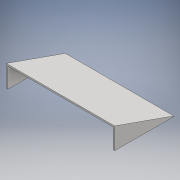
# Autodesk Inventor part: Front_Chassi
Saved by Autodesk Inventor 2018.2 (Build 222227000, 227)
## iProperties
Created: 2018-08-12
Part Number: Front_Chassi
Material: Generic
Document SubType Name: Modeling
Designer: mateu
Density: 1 g/cm^3
Appearance: Default
Author: mateu
Autodesk Inventor part; units mm, degrees
ref_plane "YZ Plane" through (0, 0, 0) normal (1, 0, 0) x (0, 1, 0)
ref_plane "XZ Plane" through (0, 0, 0) normal (0, 1, 0) x (-1, 0, 0)
ref_plane "XY Plane" through (0, 0, 0) normal (0, 0, 1) x (1, 0, 0)
sketch "Sketch1" plane through (0, 0, 0) normal (0, 0, 1) x (1, 0, 0)
  line L0 (0, 0) -> (0, 85)
  line L1 (0, 85) -> (156, 85)
  line L2 (156, 85) -> (156, 0)
  line L3 (156, 0) -> (153.6, 0)
  line L4 (153.6, 0) -> (153.6, 82.6)
  line L5 (153.6, 82.6) -> (2.4, 82.6)
  line L6 (2.4, 82.6) -> (2.4, 0)
  line L7 (2.4, 0) -> (0, 0)
  dimension "d0" = 85
  dimension "d1" = 156
  dimension "d2" = 2.4
  dimension "d3" = 82.6
  dimension "d4" = 151.2
  constraints: 16 end point, 6 perpendicular, 1 parallel, 1 point on line, 1 vertical
  measures "d0" distance of L0.start L0.end
  measures "d1" distance of L0.end L1.end
  measures "d2" distance of L2.end L3.end
  measures "d3" distance of L3.end L4.end
  measures "d4" distance of L4.end L5.end
extrude "Extrusion1" add sketch "Sketch1" along normal blind 0.9
sketch "Sketch2" plane through (0, 0, 0) normal (-1, 0, 0) x (0, 0, 1)
  line L0 (0, 0) -> (0.9, 0) projected
  line L1 (0.9, 0) -> (30.9, 0)
  line L2 (0.9, 0) -> (0.9, 85) projected
  line L3 (30.9, 0) -> (0.9, 85)
  line L4 (0.9, 85) -> (0.9, 0)
  dimension "d7" = 30
  constraints: 6 end point, 1 horizontal, 1 perpendicular
  measures "d7" distance of L0.end L1.end
extrude "Extrusion2" add sketch "Sketch2" against normal blind 2.4
sketch "Sketch3" plane through (156, 0, 0) normal (1, 0, 0) x (0, 0, -1)
  line L0 (-0.9, 0) -> (-0.9, 85) projected
  line L1 (-0.9, 0) -> (-30.8653, 0)
  line L2 (0, 0) -> (-30.9, 0) projected
  line L3 (-0.9, 0) -> (-30.9, 0)
  line L4 (0, 85) -> (-0.9, 85) projected
  line L5 (-30.9, 0) -> (-0.9, 85)
  line L6 (-0.9, 85) -> (-0.9, 0)
  constraints: 8 end point, 1 collinear, 1 horizontal, 1 perpendicular
extrude "Extrusion3" add sketch "Sketch3" against normal blind 2.4
sketch "Sketch4" plane through (2.4, 0, 0) normal (1, 0, 0) x (0, 0, -1)
  line L0 (0, 0) -> (-30.9, 0) projected
  line L1 (-30.9, 0) -> (-28.5, 0)
  line L2 (0, 82.5887) -> (0, 81.2786)
  line L3 (0, 82.6) -> (0, 0) projected
  line L4 (0, 81.2786) -> (-28.5, 0)
  line L5 (-30.9, 0) -> (-0.9, 85)
  line L6 (-0.9, 85) -> (-0.9, 82.6)
  line L7 (0, 82.6) -> (-0.9, 82.6) projected
  line L8 (-0.9, 82.6) -> (0, 82.6)
  dimension "d12" = 2.4
  constraints: 12 end point, 2 point on line, 1 collinear, 1 vertical
  measures "d12" distance of L0.end L1.end
extrude "Extrusion4" add sketch "Sketch4" along normal blind 152 contours L0 L5 L6 L7 L3 L2 L4
body "Solid1"
